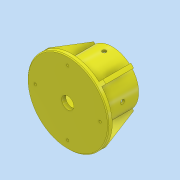
# Autodesk Inventor part: ground_support_1
Saved by Autodesk Inventor 2022 (Build 260153000, 153)
## iProperties
Created: 2019-12-20
Part Number: ground_support_1
Material: Generic
Document SubType Name: Modeling
Designer: nnico
Density: 1 g/cm^3
Appearance: Yellow
Author: nnico
Autodesk Inventor part; units mm, degrees
ref_plane "YZ Plane" through (0, 0, 0) normal (1, 0, 0) x (0, 1, 0)
ref_plane "XZ Plane" through (0, 0, 0) normal (0, 1, 0) x (-1, 0, 0)
ref_plane "XY Plane" through (0, 0, 0) normal (0, 0, 1) x (1, 0, 0)
sketch "Sketch1" plane through (0, 0, 0) normal (0, 1, 0) x (-1, 0, 0)
  circle A0 centre (0, 0) radius 50
  dimension "d0" = 100
  constraints: 1 centre point, 1 coincident
  measures "d0" diameter of A0
extrude "Extrusion1" add sketch "Sketch1" along normal blind 5
sketch "Sketch2" plane through (0, 5, 0) normal (0, 1, 0) x (1, 0, 0)
  circle A0 centre (0, 0) radius 40 construction
  line L0 (0, 40) -> (0, -40) construction
  line L1 (-40, 0) -> (40, 0) construction
  circle A1 centre (0, 40) radius 1.5
  circle A2 centre (-40, 0) radius 1.5
  circle A3 centre (0, -40) radius 1.5
  circle A4 centre (40, 0) radius 1.5
  circle A5 centre (0, 0) radius 7.5
  dimension "d3" = 80
  dimension "d4" = 3
  dimension "d5" = 3
  dimension "d6" = 3
  dimension "d7" = 3
  dimension "d10" = 15
  constraints: 6 centre point, 6 coincident, 4 end point, 4 point on circle, 3 midpoint, 1 perpendicular, 1 vertical
  measures "d3" diameter of A0
  measures "d4" diameter of A1
  measures "d5" diameter of A2
  measures "d6" diameter of A3
  measures "d7" diameter of A4
  measures "d10" diameter of A5
extrude "Extrusion2" cut sketch "Sketch2" against normal blind 5
sketch "Sketch3" plane through (0, 5, 0) normal (0, 1, 0) x (1, 0, 0)
  circle A0 centre (0, 0) radius 30.1625
  circle A1 centre (0, 0) radius 32.6625
  dimension "d11" = 60.325
  dimension "d12" = 65.325
  constraints: 2 centre point, 2 coincident
  measures "d11" diameter of A0
  measures "d12" diameter of A1
extrude "Extrusion3" add sketch "Sketch3" along normal blind 50
sketch "Sketch4" plane through (0, 5, 0) normal (0, 1, 0) x (1, 0, 0)
  circle A0 centre (0, 0) radius 50 construction
  line L0 (-50, 0) -> (50, 0) construction
  line L1 (0, -50) -> (0, 50) construction
  line L2 (-35.3553, -35.3553) -> (35.3553, 35.3553) construction
  line L3 (35.3553, -35.3553) -> (-35.3553, 35.3553) construction
  line L4 (21.1632, -17.6277) -> (37.0789, -33.5434)
  circle A1 centre (0, 0) radius 27.543 construction
  line L5 (17.6277, -21.1632) -> (33.5434, -37.0789)
  circle A2 centre (0, 0) radius 32.6625 projected
  arc A3 (21.2604, -24.7959) -> (24.7959, -21.2604) centre (0, 0) ccw
  arc A4 (33.5434, -37.0789) -> (37.0789, -33.5434) centre (0, 0) ccw
  line L6 (-21.1632, -17.6277) -> (-37.0789, -33.5434)
  line L7 (-17.6277, -21.1632) -> (-33.5434, -37.0789)
  arc A5 (-24.7959, -21.2604) -> (-21.2604, -24.7959) centre (0, 0) ccw
  arc A6 (-37.0789, -33.5434) -> (-33.5434, -37.0789) centre (0, 0) ccw
  line L8 (21.1632, 17.6277) -> (37.0789, 33.5434)
  line L9 (17.6277, 21.1632) -> (33.5434, 37.0789)
  arc A7 (24.7959, 21.2604) -> (21.2604, 24.7959) centre (0, 0) ccw
  arc A8 (37.0789, 33.5434) -> (33.5434, 37.0789) centre (0, 0) ccw
  line L10 (-17.6277, 21.1632) -> (-33.5434, 37.0789)
  line L11 (-21.1632, 17.6277) -> (-37.0789, 33.5434)
  arc A9 (-33.5434, 37.0789) -> (-37.0789, 33.5434) centre (0, 0) ccw
  arc A10 (-21.2604, 24.7959) -> (-24.7959, 21.2604) centre (0, 0) ccw
  dimension "d15" = 45
  dimension "d16" = 45
  dimension "d19" = 5
  constraints: 24 end point, 20 symmetric about line, 19 point on circle, 8 centre point, 8 point on line, 7 midpoint, 1 coincident, 1 parallel, 1 vertical, 19 other
  measures "d15" angle of L2 L1
  measures "d16" angle of L1 L3
  measures "d19" distance between parallel lines of L7 L6
extrude "Extrusion4" add sketch "Sketch4" along normal up to surface (50 mm away) contours L4 A4 L5 A2 | L7 A6 L6 A2 | A2 L9 A8 L8 | L11 A9 L10 A2
chamfer "Chamfer1" distance 45 distance2 15 1 edges at (-35.3553, 55, -35.3553) measured on face at (-35.3553, 54.5, -35.3553)
chamfer "Chamfer2" distance 45 distance2 15 1 edges at (-35.3553, 55, 35.3553) measured on face at (-35.3553, 54.5, 35.3553)
chamfer "Chamfer3" distance 45 distance2 15 1 edges at (35.3553, 55, 35.3553) measured on face at (35.3553, 54.5, 35.3553)
chamfer "Chamfer4" distance 45 distance2 15 1 edges at (35.3553, 55, -35.3553) measured on face at (35.3553, 54.5, -35.3553)
chamfer "Chamfer5" distance 1 angle 45 1 edges at (50, 0, 0)
sketch "Sketch6" plane through (0, 0, 0) normal (1, 0, 0) x (0, 1, 0)
  circle A0 centre (35, 0) radius 2.5
  line L0 (55, 30.1625) -> (55, -30.1625) projected
  point P0 (0, 0)
  dimension "d35" = 5
  dimension "d36" = 20
  constraints: 1 centre point
  measures "d35" diameter of A0
  measures "d36" distance from line of L0 A0.centre
extrude "Extrusion5" cut sketch "Sketch6" along normal through all both and the other way through all
sketch "Sketch7" plane through (0, 0, 0) normal (0, 0, 1) x (1, 0, 0)
  circle A0 centre (0, 45) radius 2.5
  line L0 (-30.1625, 55) -> (30.1625, 55) projected
  point P0 (0, 0)
  dimension "d39" = 5
  dimension "d40" = 10
  constraints: 1 centre point
  measures "d39" diameter of A0
  measures "d40" distance from line of L0 A0.centre
extrude "Extrusion6" cut sketch "Sketch7" along normal through all both and the other way through all
body "Solid1"
